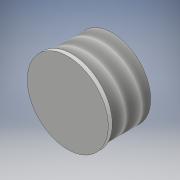
# Autodesk Inventor part: Plug
Saved by Autodesk Inventor 2017 (Build 210142000, 142)
## iProperties
Created: 2017-04-06
Part Number: Plug
Material: Generic
Document SubType Name: Modeling
Designer: AlexS
Density: 1 g/cm^3
Appearance: Default
Author: AlexS
Autodesk Inventor part; units mm, degrees
ref_plane "YZ Plane" through (0, 0, 0) normal (1, 0, 0) x (0, 1, 0)
ref_plane "XZ Plane" through (0, 0, 0) normal (0, 1, 0) x (-1, 0, 0)
ref_plane "XY Plane" through (0, 0, 0) normal (0, 0, 1) x (1, 0, 0)
sketch "Sketch2" plane through (0, 0, 0) normal (0, 0, 1) x (1, 0, 0)
  line L0 (0, 0) -> (0, 11)
  line L1 (0, 0) -> (10, 0)
  line L2 (10, 0) -> (10, 1)
  line L3 (10, 1) -> (9.5, 1)
  line L4 (9.5, 1) -> (9.5, 11)
  line L5 (9.5, 11) -> (0, 11)
  dimension "d0" = 11
  dimension "d1" = 10
  dimension "d2" = 0.5
  dimension "d3" = 1
  constraints: 12 end point, 3 perpendicular, 2 vertical, 1 horizontal
  measures "d0" distance of L0.start L0.end
  measures "d1" distance of L0.start L1.end
  measures "d2" distance of L2.end L3.end
  measures "d3" distance between parallel lines of L1 L3
revolve "Revolution1" add sketch "Sketch2" angle 360 about axis through (0, 0, 0) along (0, 1, 0)
thread "Thread1" size "M39x4" class "6g" standard "ANSI Metric M Profile" full length
body "Solid1"
